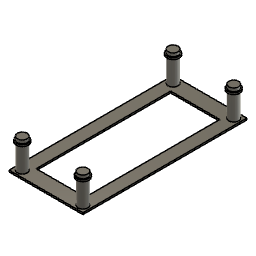
speaker_holder (Autodesk Fusion 360 design; units mm, degrees)
Autodesk Fusion 360 part; units mm, degrees
sketch "Sketch1" plane through (0, 0, 0) normal (0, 1, 0) x (1, 0, 0)
  line L0 (22.5, 50) -> (-22.5, 50)
  line L1 (-22.5, 50) -> (-22.5, -50)
  line L2 (-22.5, -50) -> (22.5, -50)
  line L3 (22.5, -50) -> (22.5, 50)
  line L4 (22.5, 50) -> (-22.5, -50) construction
  line L5 (-22.5, 50) -> (22.5, -50) construction
  line L6 (15, 41) -> (-15, 41)
  line L7 (-15, 41) -> (-15, -41)
  line L8 (-15, -41) -> (15, -41)
  line L9 (15, -41) -> (15, 41)
  line L10 (15, 41) -> (-15, -41) construction
  line L11 (-15, 41) -> (15, -41) construction
  dimension "d1" = 45
  dimension "d2" = 100
  dimension "d3" = 30
  dimension "d4" = 82
  constraint horizontal L0
  constraint perpendicular L0 L1
  constraint parallel L0 L2
  constraint parallel L1 L3
  constraint coincident L4 origin
  constraint coincident L5 origin
  constraint horizontal L6
  constraint perpendicular L6 L7
  constraint parallel L6 L8
  constraint parallel L7 L9
  constraint coincident L10 origin
  constraint coincident L11 origin
  measures "d1" distance of L1.end L2.end
  measures "d2" distance of L0.end L1.end
  measures "d3" distance of L7.end L8.end
  measures "d4" distance of L6.end L7.end
extrude "Extrude1" add sketch "Sketch1" along normal blind 1
sketch "Sketch2" plane through (0, 1, 0) normal (0, 1, 0) x (-1, 0, 0)
  line L0 (-15, -41) -> (-15, 41)
  line L1 (-15, 41) -> (15, 41)
  line L2 (15, 41) -> (15, -41)
  line L3 (15, -41) -> (-15, -41)
  line L4 (-22.5, 50) -> (-22.5, -50)
  line L5 (-22.5, -50) -> (22.5, -50)
  line L6 (22.5, -50) -> (22.5, 50)
  line L7 (22.5, 50) -> (-22.5, 50)
  circle A0 centre (18.5, -46) radius 3
  circle A1 centre (-18.5, -46) radius 3
  circle A2 centre (-18.5, 46) radius 3
  circle A3 centre (18.5, 46) radius 3
  dimension "d7" = 6
  dimension "d8" = 4
  dimension "d9" = 4
  dimension "d10" = 6
  dimension "d11" = 4
  dimension "d12" = 4
  dimension "d13" = 6
  dimension "d14" = 4
  dimension "d15" = 4
  dimension "d16" = 6
  dimension "d17" = 4
  dimension "d18" = 4
  measures "d7" diameter of A0
  measures "d8" distance of L5 A0.centre
  measures "d9" distance of L6 A0.centre
  measures "d10" diameter of A1
  measures "d11" distance of L5 A1.centre
  measures "d12" distance of L4 A1.centre
  measures "d13" diameter of A2
  measures "d14" distance of L4 A2.centre
  measures "d15" distance of L7 A2.centre
  measures "d16" diameter of A3
  measures "d17" distance of L6 A3.centre
  measures "d18" distance of L7 A3.centre
extrude "Extrude2" add sketch "Sketch2" along normal blind 15 contours A0 | A1 | A2 | A3
sketch "Sketch3" plane through (0, 16, 0) normal (0, 1, 0) x (-1, 0, 0)
  circle A0 centre (18.5, -46) radius 3
  circle A1 centre (18.5, -46) radius 3.75
  circle A2 centre (-18.5, -46) radius 3.75
  circle A3 centre (-18.5, -46) radius 3
  circle A4 centre (18.5, 46) radius 3.75
  circle A5 centre (18.5, 46) radius 3
  circle A6 centre (-18.5, 46) radius 3.75
  circle A7 centre (-18.5, 46) radius 3
  dimension "d21" = 7.5
  dimension "d22" = 7.5
  dimension "d23" = 7.5
  dimension "d24" = 7.5
  constraint concentric A0 A1
  constraint concentric A2 A3
  constraint concentric A4 A5
  constraint concentric A6 A7
  measures "d21" diameter of A1
  measures "d22" diameter of A2
  measures "d23" diameter of A4
  measures "d24" diameter of A6
extrude "Extrude3" add sketch "Sketch3" along normal blind 1 contours A0 | A1 | A2 | A3 | A4 | A5 | A6 | A7
sketch "Sketch4" plane through (0, 17, 0) normal (0, 1, 0) x (-1, 0, 0)
  circle A0 centre (-18.5, -46) radius 3.75
  circle A1 centre (-18.5, -46) radius 3
  circle A2 centre (18.5, -46) radius 3
  circle A3 centre (18.5, -46) radius 3.75
  circle A4 centre (-18.5, 46) radius 3
  circle A5 centre (-18.5, 46) radius 3.75
  circle A6 centre (18.5, 46) radius 3
  circle A7 centre (18.5, 46) radius 3.75
  dimension "d27" = 6
  dimension "d28" = 6
  dimension "d29" = 6
  dimension "d30" = 6
  constraint concentric A0 A1
  constraint concentric A2 A3
  constraint concentric A4 A5
  constraint concentric A6 A7
  measures "d27" diameter of A1
  measures "d28" diameter of A2
  measures "d29" diameter of A4
  measures "d30" diameter of A6
extrude "Extrude4" add sketch "Sketch4" along normal blind 2 contours A1 | A2 | A4 | A6
